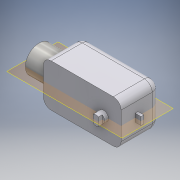
# Autodesk Inventor part: Lifting Motor
Saved by Autodesk Inventor 2016 (Build 200138000, 138)
## iProperties
Created: 2016-05-08
Part Number: Lifting Motor
Material: Generic
Document SubType Name: Modeling
Designer: Kenneth Daniel
Density: 1 g/cm^3
Appearance: Default
Author: Kenneth Daniel
Autodesk Inventor part; units mm, degrees
ref_plane "YZ Plane" through (0, 0, 0) normal (1, 0, 0) x (0, 1, 0)
ref_plane "XZ Plane" through (0, 0, 0) normal (0, 1, 0) x (-1, 0, 0)
ref_plane "XY Plane" through (0, 0, 0) normal (0, 0, 1) x (1, 0, 0)
sketch "Sketch1" plane through (0, 0, 0) normal (0, 1, 0) x (-1, 0, 0)
  line L0 (-20, 11) -> (20, 11)
  line L1 (20, 11) -> (20, -11)
  line L2 (20, -11) -> (-20, -11)
  line L3 (-20, -11) -> (-20, 11)
  line L4 (-20, 11) -> (20, -11) construction
  line L5 (20, 11) -> (-20, -11) construction
  point P0 (0, 0)
  dimension "d0" = 40
  dimension "d1" = 22
  constraints: 12 end point, 2 midpoint, 2 parallel, 1 horizontal, 1 perpendicular
  measures "d0" distance of L0.start L0.end
  measures "d1" distance of L0.end L1.end
extrude "Extrusion1" add sketch "Sketch1" along normal blind 20
fillet "Fillet1" radius 4 8 edges at (0, 20, 11) (20, 20, 0) (20, 10, 11) (20, 10, -11) (0, 20, -11) (-20, 10, -11) (-20, 20, 0) (-20, 10, 11)
sketch "Sketch2" plane through (20, 0, 7) normal (1, 0, 0) x (0, 0, -1)
  line L0 (14, 0) -> (0, 0) construction
  line L1 (14, 16) -> (18, 16) construction
  line L2 (0, 0) -> (14, 16) construction
  line L3 (14, 16) -> (0, 16) construction
  line L4 (0, 16) -> (14, 0) construction
  line L5 (9, 8.75) -> (5, 8.75)
  line L6 (5, 8.75) -> (5, 7.25)
  line L7 (5, 7.25) -> (9, 7.25)
  line L8 (9, 7.25) -> (9, 8.75)
  line L9 (9, 8.75) -> (5, 7.25) construction
  line L10 (5, 8.75) -> (9, 7.25) construction
  point P0 (7, 0)
  point P1 (7, 8)
  dimension "d5" = 4
  dimension "d6" = 1.5
  constraints: 18 end point, 3 midpoint, 2 parallel, 1 collinear, 1 horizontal, 1 perpendicular
  measures "d5" distance of L5.start L5.end
  measures "d6" distance of L6.end L5.end
extrude "Extrusion2" add sketch "Sketch2" along normal blind 3
sketch "Sketch3" plane through (0, 0, 0) normal (0, -1, 0) x (1, 0, 0)
  arc A0 (20, 7) -> (16, 11) centre (16, 7) ccw projected
  arc A1 (-20, -7) -> (-16, -11) centre (-16, -7) ccw projected
  line L0 (16, 7) -> (-16, -7) construction
  line L1 (-16, 7) -> (-16, 11) projected
  line L2 (-16, -7) -> (-16, 7) construction
  line L3 (20, -7) -> (16, -7) projected
  line L4 (-16, 7) -> (16, -7) construction
  line L5 (16, -7) -> (16, 7) construction
  line L6 (16, 7) -> (11, 7) construction
  line L7 (16, 7) -> (-16, 7) construction
  line L8 (11, 7) -> (11, -7) construction
  circle A2 centre (11, 0) radius 2.5
  point P0 (0, 0)
  dimension "d9" = 5
  dimension "d10" = 5
  constraints: 10 end point, 1 centre point, 1 collinear, 1 midpoint, 1 perpendicular, 1 point on line
  measures "d9" distance of L0.start L6.end
  measures "d10" diameter of A2
extrude "Extrusion3" add sketch "Sketch3" along normal blind 2
sketch "Sketch4" plane through (11, -2, 0) normal (0, -1, 0) x (1, 0, 0)
  line L0 (-1.3, -4.4849) -> (1.3, -4.4849)
  line L1 (1.3, -2.1354) -> (1.3, 2.1354)
  line L2 (-1.3, 2.1354) -> (-1.3, -2.1354)
  line L3 (-1.3, -4.4849) -> (1.3, 4.4849) construction
  line L4 (1.3, -4.4849) -> (-1.3, 4.4849) construction
  circle A0 centre (0, 0) radius 2.5 projected
  arc A1 (1.3, 2.1354) -> (-1.3, 2.1354) centre (0, 0) ccw
  arc A2 (-1.3, -2.1354) -> (1.3, -2.1354) centre (0, 0) ccw
  point P0 (-11, 0)
  dimension "d13" = 2.6
  constraints: 10 end point, 4 point on circle, 2 centre point, 2 midpoint, 1 coincident, 1 horizontal, 1 parallel, 1 perpendicular
  measures "d13" distance of L0.start L0.end
extrude "Extrusion4" add sketch "Sketch4" along normal blind 2 contours A0 L2 L1
sketch "Sketch5" plane through (-20, 0, -7) normal (-1, 0, 0) x (0, 0, 1)
  line L0 (5, 8.75) -> (9, 8.75) projected
  circle A0 centre (7, 8.75) radius 7.0401
  point P0 (7, 0)
  constraints: 1 centre point, 1 midpoint
extrude "Extrusion5" add sketch "Sketch5" along normal blind 11
ref_plane "Work Plane1" through (-16, 0, 0) normal (0, 0, 1) x (1, 0, 0)
body "Solid1"
